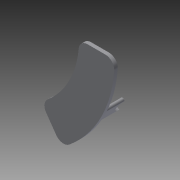
# Autodesk Inventor part: spoelhouder
Saved by Autodesk Inventor 2014 (Build 180170000, 170)
## iProperties
Created: 2015-03-19
Part Number: spoelhouder
Material: Generic
Document SubType Name: Modeling
Designer: MSI
Density: 1 g/cm^3
Appearance: Default
Author: MSI
Autodesk Inventor part; units mm, degrees
ref_plane "YZ Plane" through (0, 0, 0) normal (1, 0, 0) x (0, 1, 0)
ref_plane "XZ Plane" through (0, 0, 0) normal (0, 1, 0) x (-1, 0, 0)
ref_plane "XY Plane" through (0, 0, 0) normal (0, 0, 1) x (1, 0, 0)
sketch "Sketch1" plane through (0, 0, 0) normal (0, 1, 0) x (-1, 0, 0)
  line L0 (0, 0) -> (-100, 0) construction
  line L1 (0, 0) -> (-57.3576, -81.9152) construction
  arc A0 (-49.793, -4.5455) -> (-32.2835, -38.1808) centre (0, 0) ccw
  arc A1 (-69.7926, -5.3846) -> (-44.4422, -54.0823) centre (0, 0) ccw
  line L2 (-54.7723, 0) -> (-64.8074, 0)
  line L3 (-31.4161, -44.8668) -> (-37.172, -53.0871)
  arc A2 (-49.793, -4.5455) -> (-54.7723, 0) centre (-54.7723, -5) ccw
  arc A3 (-64.8074, 0) -> (-69.7926, -5.3846) centre (-64.8074, -5) ccw
  arc A4 (-44.4422, -54.0823) -> (-37.172, -53.0871) centre (-41.2678, -50.2192) ccw
  arc A5 (-31.4161, -44.8668) -> (-32.2835, -38.1808) centre (-35.5118, -41.9989) ccw
  point P0 (-50, 0)
  point P1 (-28.6788, -40.9576)
  point P2 (-70, 0)
  point P3 (-40.1504, -57.3406)
  point P4 (-50, 0)
  dimension "d0" = 100
  dimension "d1" = 100
  dimension "d2" = 55
  dimension "d3" = 50
  dimension "d4" = 70
  dimension "d5" = 5
  dimension "d6" = 5
  dimension "d7" = 5
  constraints: 16 point on circle, 8 end point, 8 tangent, 6 centre point, 5 point on line, 3 midpoint, 2 coincident, 2 collinear, 1 equal radius, 1 horizontal alignment
  measures "d0" distance of L0.start L0.end
  measures "d1" distance of L0.start L1.end
  measures "d2" angle of L0 L1
  measures "d3" radius of A0
  measures "d4" radius of A1
  measures "d5" radius of A2
  measures "d6" radius of A4
  measures "d7" radius of A5
extrude "Extrusion1" add sketch "Sketch1" along normal blind 2
sketch "Sketch2" plane through (0, 2, 0) normal (0, 1, 0) x (1, 0, 0)
  arc A0 (69.7926, 5.3846) -> (44.4422, 54.0823) centre (0, 0) ccw projected
  arc A1 (49.793, 4.5455) -> (32.2835, 38.1808) centre (0, 0) ccw projected
  line L0 (0, 0) -> (62.0908, 32.3224) construction
  line L1 (0, 0) -> (70, 0) construction
  arc A2 (49.793, 4.5455) -> (54.7723, 0) centre (54.7723, 5) ccw projected
  line L2 (54.7723, 0) -> (64.8074, 0) projected
  arc A3 (64.8074, 0) -> (69.7926, 5.3846) centre (64.8074, 5) ccw projected
  arc A4 (69.7926, 5.3846) -> (44.4422, 54.0823) centre (0, 0) ccw projected
  arc A5 (44.4422, 54.0823) -> (37.172, 53.0871) centre (41.2678, 50.2192) ccw projected
  line L3 (37.172, 53.0871) -> (31.4161, 44.8668) projected
  arc A6 (31.4161, 44.8668) -> (32.2835, 38.1808) centre (35.5118, 41.9989) ccw projected
  arc A7 (49.793, 4.5455) -> (32.2835, 38.1808) centre (0, 0) ccw projected
  line L4 (44.3505, 23.0874) -> (46.1975, 19.5394)
  line L5 (46.1975, 19.5394) -> (63.8363, 28.7215)
  line L6 (63.8363, 28.7215) -> (61.9893, 32.2696)
  line L7 (44.3505, 23.0874) -> (42.5035, 26.6355)
  line L8 (42.5035, 26.6355) -> (60.1423, 35.8176)
  line L9 (60.1423, 35.8176) -> (61.9893, 32.2696)
  dimension "d10" = 27.5
  dimension "d12" = 4
  constraints: 16 end point, 4 point on circle, 2 perpendicular, 2 symmetric about line, 2 tangent, 1 equal length, 1 horizontal, 1 point on line
  measures "d10" angle of L1 L0
  measures "d12" distance of L4.start L4.end
extrude "Extrusion2" add sketch "Sketch2" along normal blind 10 contours L5 L4 L7 L8 L9 L6
sketch "Sketch3" plane through (60.1423, 2, -35.8176) normal (0.8870108, 0, -0.4617486) x (-0.4617486, 0, -0.8870108)
  line L0 (-8, 10) -> (0, 10) projected
  circle A0 centre (-4, 9.5) radius 3
  point P0 (-4, -2)
  point P1 (-4, 10)
  dimension "d17" = 6
  dimension "d18" = 0.5
  constraints: 1 centre point, 1 midpoint, 1 vertical alignment
  measures "d17" diameter of A0
  measures "d18" distance from line of L0 A0.centre
extrude "Extrusion3" cut sketch "Sketch3" against normal blind 20
sketch "Sketch4" plane through (0, 12, 0) normal (0, 1, 0) x (1, 0, 0)
  line L0 (46.1975, 19.5394) -> (63.8363, 28.7215) projected
  line L1 (42.9847, 25.7112) -> (60.6234, 34.8934) projected
  line L2 (60.6234, 34.8934) -> (60.1423, 35.8176) projected
  line L3 (60.1423, 35.8176) -> (42.5035, 26.6355) projected
  line L4 (42.5035, 26.6355) -> (42.9847, 25.7112) projected
  line L5 (63.3552, 29.6458) -> (45.7164, 20.4636) projected
  line L6 (60.6234, 34.8934) -> (63.3552, 29.6458) projected
  line L7 (42.9847, 25.7112) -> (60.6234, 34.8934) projected
  line L8 (45.7164, 20.4636) -> (42.9847, 25.7112) projected
  line L9 (44.1761, 27.5062) -> (47.8701, 20.4101)
  line L10 (58.3683, 34.8941) -> (62.0623, 27.798)
  point P0 (0, 0)
  dimension "d21" = 2
  dimension "d22" = 16
  constraints: 4 end point, 4 point on line, 2 perpendicular
  measures "d21" distance between parallel lines of L6 L10
  measures "d22" distance between parallel lines of L10 L9
extrude "Extrusion4" cut sketch "Sketch4" against normal blind 10 contours L9 L5 L10 L0 | L9 L1 L10 L5 | L9 L3 L10 L1
fillet "Fillet1" radius 1 8 edges at (63.8363, 7, -28.7215) (62.0623, 7, -27.798) (60.1423, 7, -35.8176) (58.3683, 7, -34.8941) (44.1761, 7, -27.5062) (42.5035, 7, -26.6355) (47.8701, 7, -20.4101) (46.1975, 7, -19.5394)
body "Solid1"
